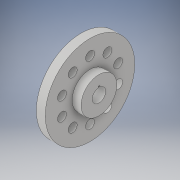
# Autodesk Inventor part: arthurWeiActivity 5.5a#4.dwg
Saved by Autodesk Inventor 2018 (Build 220112000, 112)
## iProperties
Created: 2019-01-15
Part Number: arthurWeiActivity 5.5a#4.dwg
Material: Generic
Document SubType Name: Modeling
Designer: This kid
Density: 1 g/cm^3
Appearance: Default
Author: This kid
Autodesk Inventor part; units mm, degrees
ref_plane "YZ Plane" through (0, 0, 0) normal (1, 0, 0) x (0, 1, 0)
ref_plane "XZ Plane" through (0, 0, 0) normal (0, 1, 0) x (-1, 0, 0)
ref_plane "XY Plane" through (0, 0, 0) normal (0, 0, 1) x (1, 0, 0)
sketch "Sketch1" plane through (0, 0, 0) normal (0, 0, 1) x (1, 0, 0)
  line L0 (-2.7173, 13.7894) -> (9.9827, 13.7894)
  line L1 (9.9827, 13.7894) -> (9.9827, -24.3106)
  line L2 (9.9827, -40.1856) -> (-2.7173, -40.1856)
  line L3 (-2.7173, -40.1856) -> (-2.7173, 13.7894)
  line L4 (-2.7173, -40.1856) -> (22.6827, -40.1856)
  line L5 (22.6827, -40.1856) -> (22.6827, -24.3106)
  line L6 (22.6827, -24.3106) -> (9.9827, -24.3106)
  line L7 (-2.7173, -24.3106) -> (-2.7173, -40.1856)
  line L8 (-16.1487, -49.7106) -> (31.6829, -49.7106)
  point P0 (0, 0)
  dimension "d0" = 12.7
  dimension "d1" = 53.975
  dimension "d4" = 25.4
  dimension "d5" = 15.875
  dimension "d6" = 9.525
  constraints: 18 end point, 4 parallel, 3 horizontal, 2 perpendicular
  measures "d0" distance of L2.start L2.end
  measures "d1" distance of L0.end L2.start
  measures "d4" distance of L7.start L5.end
  measures "d5" distance of L5.end L4.end
  measures "d6" distance between parallel lines of L8 L4
revolve "Revolution1" add sketch "Sketch1" angle 360 about axis through (-16.1487, -49.7106, 0) along (1, 0, 0)
sketch "Sketch3" plane through (22.6827, -49.7106, 0) normal (1, 0, 0) x (0, 0, -1)
  line L0 (0, 11.43) -> (-1.27, 11.43)
  line L1 (0, 11.43) -> (1.27, 11.43)
  line L2 (1.27, 11.43) -> (1.27, 9.44)
  circle A0 centre (0, 0) radius 9.525 projected
  line L3 (-1.27, 11.43) -> (-1.27, 9.44)
  line L4 (1.27, 9.44) -> (-1.27, 9.44)
  point P0 (0, 49.7106)
  dimension "d9" = 1.27
  dimension "d10" = 1.27
  constraints: 10 end point, 2 point on circle, 1 horizontal, 1 parallel, 1 perpendicular
  measures "d9" distance of L0.start L0.end
  measures "d10" distance of L0.start L1.end
extrude "Extrusion1" cut sketch "Sketch3" against normal blind 25.4 contours L1 L2 A0 L3 L0
sketch "Sketch7" plane through (22.6827, -49.7106, 0) normal (1, 0, 0) x (0, 0, -1)
  point P0 (0, 49.7106)
  point P1 (0, 0)
  point P2 (0, 41.91)
  point P3 (-24.6341, 33.9059)
  point P4 (-39.8588, 12.9509)
  point P5 (-39.8588, -12.9509)
  point P6 (-24.6341, -33.9059)
  point P7 (0, -41.91)
  point P8 (24.6341, -33.9059)
  point P9 (39.8588, -12.9509)
  point P10 (39.8588, 12.9509)
  point P11 (24.6341, 33.9059)
  dimension "d29" = 41.91
  dimension "d32" = 360
  constraints: 11 other
  measures "d29" distance of point (0, 41.91) point (0, 0)
hole "Hole3" at (22.6827, -49.7106, 0) at (22.6827, -7.8006, 0) at (22.6827, -15.8047, 24.6341) at (22.6827, -36.7597, 39.8588) at (22.6827, -62.6615, 39.8588) at (22.6827, -83.6165, 24.6341) at (22.6827, -91.6206, 0) at (22.6827, -83.6165, -24.6341) at (22.6827, -62.6615, -39.8588) at (22.6827, -36.7597, -39.8588) at (22.6827, -15.8047, -24.6341) direction (-1, 0, 0) diameter 12.7 end through all
body "Solid1"
